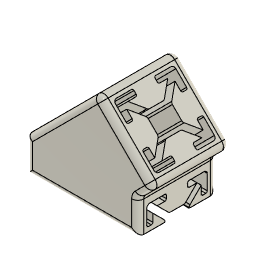
45base_new v6 (Autodesk Fusion 360 design; units mm, degrees)
Autodesk Fusion 360 part; units mm, degrees
sketch "Sketch1" plane through (0, 0, 0) normal (0, 0, 1) x (1, 0, 0)
sketch "Sketch2" plane through (0, 0, 0) normal (0, 0, 1) x (1, 0, 0)
  line L0 (-9, -10) -> (-4, -10)
  arc A0 (-4, -10) -> (-3.5, -9.5) centre (-4, -9.5) ccw
  line L1 (-3.5, -9.5) -> (-3.5, -8.5)
  arc A1 (-3.5, -8.5) -> (-4, -8) centre (-4, -8.5) ccw
  line L2 (-4, -8) -> (-6.5858, -8)
  line L3 (-6.5858, -8) -> (-2.8787, -4.2929)
  arc A2 (-2.1716, -4) -> (-2.8787, -4.2929) centre (-2.1716, -5) ccw
  line L4 (-2.1716, -4) -> (2.1716, -4)
  arc A3 (2.8787, -4.2929) -> (2.1716, -4) centre (2.1716, -5) ccw
  line L5 (2.8787, -4.2929) -> (6.5858, -8)
  line L6 (6.5858, -8) -> (4, -8)
  arc A4 (4, -8) -> (3.5, -8.5) centre (4, -8.5) ccw
  line L7 (3.5, -8.5) -> (3.5, -9.5)
  arc A5 (3.5, -9.5) -> (4, -10) centre (4, -9.5) ccw
  line L8 (4, -10) -> (9, -10)
  arc A6 (9, -10) -> (10, -9) centre (9, -9) ccw
  line L9 (10, -9) -> (10, -4)
  arc A7 (10, -4) -> (9.5, -3.5) centre (9.5, -4) ccw
  line L10 (9.5, -3.5) -> (8.5, -3.5)
  arc A8 (8.5, -3.5) -> (8, -4) centre (8.5, -4) ccw
  line L11 (8, -4) -> (8, -6.5858)
  line L12 (8, -6.5858) -> (4.2929, -2.8787)
  arc A9 (4, -2.1716) -> (4.2929, -2.8787) centre (5, -2.1716) ccw
  line L13 (4, -2.1716) -> (4, 2.1753)
  arc A10 (4.2903, 2.8761) -> (4, 2.1753) centre (4.9911, 2.1753) ccw
  line L14 (4.2903, 2.8761) -> (8, 6.5858)
  line L15 (8, 6.5858) -> (8, 4)
  arc A11 (8, 4) -> (8.5, 3.5) centre (8.5, 4) ccw
  line L16 (8.5, 3.5) -> (9.5, 3.5)
  arc A12 (9.5, 3.5) -> (10, 4) centre (9.5, 4) ccw
  line L17 (10, 4) -> (10, 9)
  arc A13 (10, 9) -> (9, 10) centre (9, 9) ccw
  line L18 (9, 10) -> (4, 10)
  arc A14 (4, 10) -> (3.5, 9.5) centre (4, 9.5) ccw
  line L19 (3.5, 9.5) -> (3.5, 8.5)
  arc A15 (3.5, 8.5) -> (4, 8) centre (4, 8.5) ccw
  line L20 (4, 8) -> (6.5858, 8)
  line L21 (6.5858, 8) -> (2.8761, 4.2903)
  arc A16 (2.1753, 4) -> (2.8761, 4.2903) centre (2.1753, 4.9911) ccw
  line L22 (2.1753, 4) -> (-2.1753, 4)
  arc A17 (-2.8761, 4.2903) -> (-2.1753, 4) centre (-2.1753, 4.9911) ccw
  line L23 (-2.8761, 4.2903) -> (-6.5858, 8)
  line L24 (-6.5858, 8) -> (-4, 8)
  arc A18 (-4, 8) -> (-3.5, 8.5) centre (-4, 8.5) ccw
  line L25 (-3.5, 8.5) -> (-3.5, 9.5)
  arc A19 (-3.5, 9.5) -> (-4, 10) centre (-4, 9.5) ccw
  line L26 (-4, 10) -> (-9, 10)
  arc A20 (-9, 10) -> (-10, 9) centre (-9, 9) ccw
  line L27 (-10, 9) -> (-10, 4)
  arc A21 (-10, 4) -> (-9.5, 3.5) centre (-9.5, 4) ccw
  line L28 (-9.5, 3.5) -> (-8.5, 3.5)
  arc A22 (-8.5, 3.5) -> (-8, 4) centre (-8.5, 4) ccw
  line L29 (-8, 4) -> (-8, 6.5858)
  line L30 (-8, 6.5858) -> (-4.2929, 2.8787)
  arc A23 (-4, 2.1716) -> (-4.2929, 2.8787) centre (-5, 2.1716) ccw
  line L31 (-4, 2.1716) -> (-4, -2.1716)
  arc A24 (-4.2929, -2.8787) -> (-4, -2.1716) centre (-5, -2.1716) ccw
  line L32 (-4.2929, -2.8787) -> (-8, -6.5858)
  line L33 (-8, -6.5858) -> (-8, -4)
  arc A25 (-8, -4) -> (-8.5, -3.5) centre (-8.5, -4) ccw
  line L34 (-8.5, -3.5) -> (-9.5, -3.5)
  arc A26 (-9.5, -3.5) -> (-10, -4) centre (-9.5, -4) ccw
  line L35 (-10, -4) -> (-10, -9)
  arc A27 (-10, -9) -> (-9, -10) centre (-9, -9) ccw
  circle A28 centre (0, 0) radius 2
  line L36 (-13, 13) -> (13, 13)
  line L37 (13, 13) -> (13, -13)
  line L38 (13, -13) -> (-13, -13)
  line L39 (-13, -13) -> (-13, 13)
  line L40 (-13, 13) -> (13, -13) construction
  line L41 (13, 13) -> (-13, -13) construction
  dimension "d1" = 26
  dimension "d2" = 26
  constraint horizontal L36
  constraint perpendicular L36 L37
  constraint parallel L36 L38
  constraint parallel L37 L39
  constraint coincident L40 A28.centre
  constraint coincident L41 A28.centre
  constraint coincident A28.centre origin
  measures "d1" distance of L37.end L38.end
  measures "d2" distance of L36.end L37.end
extrude "Extrude1" add sketch "Sketch2" along normal blind 40 contours L36 L37 L38 L39 makes body 1
scale "Scale1" factor 1.2 about (4, 2.1753, 40) bodies 1
move_body "Move1" bodies 1 to x (1, 0, 0) y (0, 0.707107, 0.707107) z (0, -0.707107, 0.707107) at (0, 11.7432, 1.5546)
copy_body "CopyPasteBodies1" bodies 1 makes body 2
move_body "Move2" bodies 2 to x (1, 0, 0) y (0, 0.707107, 0.707107) z (0, -0.707107, 0.707107) at (0, 8.9174, 3.5928)
move_body "Move3" bodies 2 to x (1, 0, 0) y (0, 1, 0) z (0, 0, 1) at (-39.5224, -12.7838, -23.7812)
move_body "Move4" bodies 1 to x (1, 0, 0) y (0, 1, 0) z (0, 0, 1) at (-39.5224, -42.7235, 19.8203)
extrude "Extrude2" add 1 faces at (-39.4538, -31.4911, 9.5504) along direction (0, 0.707107, -0.707107) blind 35 on bodies 1 bodies 1 2
extrude "Extrude3" cut 1 faces at (-48.6097, 11.338, -10.3518) along direction (0, -1, 0) blind 5 on bodies 1 bodies 1
extrude "Extrude4" add 1 faces at (-48.6097, 6.338, -10.3518) along direction (0, 1, 0) blind 1.123 on bodies 1 bodies 1
sketch "Sketch3" plane through (0, -36.662, 0) normal (0, -1, 0) x (1, 0, 0)
  line L0 (-49.9224, -19.1234) -> (-45.4739, -14.6749)
  arc A0 (-45.4739, -14.6749) -> (-45.1224, -13.8264) centre (-46.3224, -13.8264) ccw
  line L1 (-45.1224, -13.8264) -> (-45.1224, -8.6146)
  arc A1 (-45.1224, -8.6146) -> (-45.4739, -7.7661) centre (-46.3224, -8.6146) ccw
  line L2 (-45.4739, -7.7661) -> (-49.9224, -3.3175)
  line L3 (-49.9224, -3.3175) -> (-49.9224, -6.4205)
  arc A2 (-50.5224, -7.0205) -> (-49.9224, -6.4205) centre (-50.5224, -6.4205) ccw
  line L4 (-50.5224, -7.0205) -> (-51.7224, -7.0205)
  arc A3 (-52.3224, -6.4205) -> (-51.7224, -7.0205) centre (-51.7224, -6.4205) ccw
  line L5 (-52.3224, -6.4205) -> (-52.3224, -0.4205)
  arc A4 (-51.1224, 0.7795) -> (-52.3224, -0.4205) centre (-51.1224, -0.4205) ccw
  line L6 (-51.1224, 0.7795) -> (-45.1224, 0.7795)
  arc A5 (-44.5224, 0.1795) -> (-45.1224, 0.7795) centre (-45.1224, 0.1795) ccw
  line L7 (-44.5224, 0.1795) -> (-44.5224, -1.0205)
  arc A6 (-45.1224, -1.6205) -> (-44.5224, -1.0205) centre (-45.1224, -1.0205) ccw
  line L8 (-45.1224, -1.6205) -> (-48.2253, -1.6205)
  line L9 (-48.2253, -1.6205) -> (-43.7737, -6.0721)
  arc A7 (-43.7737, -6.0721) -> (-42.9327, -6.4205) centre (-42.9327, -5.2311) ccw
  line L10 (-42.9327, -6.4205) -> (-37.7121, -6.4205)
  arc A8 (-37.7121, -6.4205) -> (-36.8711, -6.0721) centre (-37.7121, -5.2311) ccw
  line L11 (-36.8711, -6.0721) -> (-32.4194, -1.6205)
  line L12 (-32.4194, -1.6205) -> (-35.5224, -1.6205)
  arc A9 (-36.1224, -1.0205) -> (-35.5224, -1.6205) centre (-35.5224, -1.0205) ccw
  line L13 (-36.1224, -1.0205) -> (-36.1224, 0.1795)
  arc A10 (-35.5224, 0.7795) -> (-36.1224, 0.1795) centre (-35.5224, 0.1795) ccw
  line L14 (-35.5224, 0.7795) -> (-29.5224, 0.7795)
  arc A11 (-28.3224, -0.4205) -> (-29.5224, 0.7795) centre (-29.5224, -0.4205) ccw
  line L15 (-28.3224, -0.4205) -> (-28.3224, -6.4205)
  arc A12 (-28.9224, -7.0205) -> (-28.3224, -6.4205) centre (-28.9224, -6.4205) ccw
  line L16 (-28.9224, -7.0205) -> (-30.1224, -7.0205)
  arc A13 (-30.7224, -6.4205) -> (-30.1224, -7.0205) centre (-30.1224, -6.4205) ccw
  line L17 (-30.7224, -6.4205) -> (-30.7224, -3.3175)
  line L18 (-30.7224, -3.3175) -> (-35.174, -7.7692)
  arc A14 (-35.174, -7.7692) -> (-35.5224, -8.6102) centre (-34.3331, -8.6102) ccw
  line L19 (-35.5224, -8.6102) -> (-35.5224, -13.8264)
  arc A15 (-35.5224, -13.8264) -> (-35.1709, -14.6749) centre (-34.3224, -13.8264) ccw
  line L20 (-35.1709, -14.6749) -> (-30.7224, -19.1234)
  line L21 (-30.7224, -19.1234) -> (-30.7224, -16.0205)
  arc A16 (-30.1224, -15.4205) -> (-30.7224, -16.0205) centre (-30.1224, -16.0205) ccw
  line L22 (-30.1224, -15.4205) -> (-28.9224, -15.4205)
  arc A17 (-28.3224, -16.0205) -> (-28.9224, -15.4205) centre (-28.9224, -16.0205) ccw
  line L23 (-28.3224, -16.0205) -> (-28.3224, -22.0205)
  arc A18 (-29.5224, -23.2205) -> (-28.3224, -22.0205) centre (-29.5224, -22.0205) ccw
  line L24 (-29.5224, -23.2205) -> (-35.5224, -23.2205)
  arc A19 (-36.1224, -22.6205) -> (-35.5224, -23.2205) centre (-35.5224, -22.6205) ccw
  line L25 (-36.1224, -22.6205) -> (-36.1224, -21.4205)
  arc A20 (-35.5224, -20.8205) -> (-36.1224, -21.4205) centre (-35.5224, -21.4205) ccw
  line L26 (-35.5224, -20.8205) -> (-32.4194, -20.8205)
  line L27 (-32.4194, -20.8205) -> (-36.868, -16.3719)
  arc A21 (-36.868, -16.3719) -> (-37.7165, -16.0205) centre (-37.7165, -17.2205) ccw
  line L28 (-37.7165, -16.0205) -> (-42.9283, -16.0205)
  arc A22 (-42.9283, -16.0205) -> (-43.7768, -16.3719) centre (-42.9283, -17.2205) ccw
  line L29 (-43.7768, -16.3719) -> (-48.2253, -20.8205)
  line L30 (-48.2253, -20.8205) -> (-45.1224, -20.8205)
  arc A23 (-44.5224, -21.4205) -> (-45.1224, -20.8205) centre (-45.1224, -21.4205) ccw
  line L31 (-44.5224, -21.4205) -> (-44.5224, -22.6205)
  arc A24 (-45.1224, -23.2205) -> (-44.5224, -22.6205) centre (-45.1224, -22.6205) ccw
  line L32 (-45.1224, -23.2205) -> (-51.1224, -23.2205)
  arc A25 (-52.3224, -22.0205) -> (-51.1224, -23.2205) centre (-51.1224, -22.0205) ccw
  line L33 (-52.3224, -22.0205) -> (-52.3224, -16.0205)
  arc A26 (-51.7224, -15.4205) -> (-52.3224, -16.0205) centre (-51.7224, -16.0205) ccw
  line L34 (-51.7224, -15.4205) -> (-50.5224, -15.4205)
  arc A27 (-49.9224, -16.0205) -> (-50.5224, -15.4205) centre (-50.5224, -16.0205) ccw
  line L35 (-49.9224, -16.0205) -> (-49.9224, -19.1234)
  line L36 (-55.9224, -26.8205) -> (-24.7224, -26.8205)
  line L37 (-24.7224, -26.8205) -> (-24.7224, 4.3795)
  line L38 (-24.7224, 4.3795) -> (-55.9224, 4.3795)
  line L39 (-55.9224, 4.3795) -> (-55.9224, -26.8205)
extrude "Extrude5" cut sketch "Sketch3" against normal blind 143 contours L0 A0 L1 A1 L2 L3 A2 L4 A3 L5 A4 L6 A5 L7 A6 L8 L9 A7 L10 A8 L11 L12 A9 L13 A10 L14 A11 L15 A12 L16 A13 L17 L18 A14 L19 A15 L20 L21 A16 L22 A17 L23 A18 L24 A19 L25 A20 L26 L27 A21 L28 A22 L29 L30 A23 L31 A24 L32 A25 L33 A26 L34 A27 L35 bodies 1
move_body "Move5" bodies 1 to x (1, 0, 0) y (0, 1, 0) z (0, 0, 1) at (24.7224, 14.6005, 26.8205)
move_body "Move6" bodies 1 to x (0, 1, 0) y (-1, 0, 0) z (0, 0, 1) at (-10.9279, -10.9279, 0)
move_body "Move7" bodies 1 to x (1, 0, 0) y (0, 1, 0) z (0, 0, 1) at (32.9894, 42.1279, 0)
extrude "Extrude6" cut 1 faces at (67.6475, 7.3127, 75.5578) along direction (-0.707107, 0, -0.707107) blind 38 on bodies 1 bodies 1
extrude "Extrude7" cut 1 faces at (40.7774, 7.3127, 48.6877) along direction (-0.707107, 0, -0.707107) blind 1.2 on bodies 1 bodies 1
scale "Scale2" factor 0.8333 about (0, 3.6, 20.4) bodies 1
extrude "Extrude8" cut 1 faces at (24.5118, 17.9328, 3.4007) along direction (0, 0, 1) blind 15 on bodies 1 bodies 1
fillet "Fillet1" radius 2 15 edges at (36.7677, 0.6001, 23.9002) (36.7677, 13.5996, 29.3996) (36.7677, 26.5991, 23.9002) (18.3838, 0.6001, 18.4007) (41.9529, 13.5996, 34.5849) (39.3603, 0.6001, 31.9923) (39.3603, 26.5991, 31.9923) (32.7609, 26.5991, 43.7769) (32.7609, 0.6001, 43.7769) (23.5689, 13.5996, 52.9689) (11.7843, 0.6001, 41.1843) (0, 0.6001, 23.9002) (11.7843, 26.5991, 41.1843) (0, 26.5991, 23.9002) (18.3838, 26.5991, 18.4007) on bodies 1
